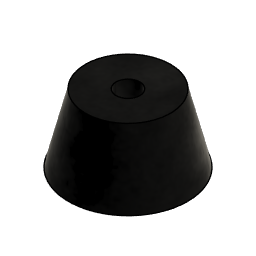
slider (Autodesk Fusion 360 archive; units mm, degrees)
design "feet"
Autodesk Fusion 360 part; units mm, degrees
sketch "Sketch1" plane through (0, 0, 0) normal (0, 0, 1) x (1, 0, 0)
  circle A0 centre (0, 0) radius 2.1
  circle A1 centre (0, 0) radius 10.5
  dimension "d1" = 4.2
  dimension "d2" = 21
  constraint coincident A0.centre A1.centre
  constraint concentric A0 A1
  measures "d1" diameter of A0
  measures "d2" diameter of A1
extrude "Extrude1" add sketch "Sketch1" along normal blind 12
chamfer "Chamfer1" distance 3 distance2 12 1 edges at (-9.7894, -3.797, 12) measured on face at (7.6609, -0.5216, 12)
